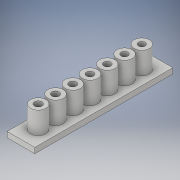
# Autodesk Inventor part: test_gwintow
Saved by Autodesk Inventor 2019 (Build 230136000, 136)
## iProperties
Created: 2019-09-16
Part Number: test_gwintow
Material: Ogólny
Document SubType Name: Modeling
Designer: mikol
Density: 1 g/cm^3
Appearance: Domyślna
Author: mikol
Autodesk Inventor part; units mm, degrees
ref_plane "YZ Plane" through (0, 0, 0) normal (1, 0, 0) x (0, 1, 0)
ref_plane "XZ Plane" through (0, 0, 0) normal (0, 1, 0) x (-1, 0, 0)
ref_plane "XY Plane" through (0, 0, 0) normal (0, 0, 1) x (1, 0, 0)
sketch "Sketch1" plane through (0, 0, 0) normal (0, 1, 0) x (-1, 0, 0)
  line L0 (5, 25) -> (-5, 25)
  line L1 (-5, 25) -> (-5, -25)
  line L2 (-5, -25) -> (5, -25)
  line L3 (5, -25) -> (5, 25)
  line L4 (5, 25) -> (-5, -25) construction
  line L5 (-5, 25) -> (5, -25) construction
  point P0 (0, 0)
  dimension "d0" = 10
  dimension "d1" = 50
  constraints: 12 end point, 2 midpoint, 2 parallel, 1 horizontal, 1 perpendicular
  measures "d0" distance of L2.end L1.end
  measures "d1" distance of L1.end L0.end
extrude "Extrusion1" add sketch "Sketch1" along normal blind 2
sketch "Sketch2" plane through (0, 2, 0) normal (0, 1, 0) x (1, 0, 0)
  circle A0 centre (0, 18.75) radius 1.2
  line L0 (5, 25) -> (-5, 25) projected
  circle A1 centre (0, 12.5) radius 1.225
  circle A2 centre (0, 6.25) radius 1.25
  circle A3 centre (0, 0) radius 1.275
  circle A4 centre (0, -6.25) radius 1.3
  circle A5 centre (0, -12.5) radius 1.325
  circle A6 centre (0, -18.75) radius 1.35
  line L1 (0, 35) -> (0, -35) projected
  line L2 (-5, -25) -> (5, -25) projected
  dimension "d4" = 2.4
  dimension "d5" = 6.25
  dimension "d6" = 2.45
  dimension "d7" = 2.5
  dimension "d8" = 2.55
  dimension "d9" = 2.6
  dimension "d10" = 2.65
  dimension "d11" = 2.7
  dimension "d12" = 6.25
  dimension "d13" = 6.25
  dimension "d14" = 6.25
  dimension "d15" = 6.25
  dimension "d17" = 6.25
  dimension "d18" = 6.25
  dimension "d19" = 6.25
  constraints: 7 centre point, 8 other
  measures "d4" diameter of A0
  measures "d5" distance from line of L0 A0.centre
  measures "d6" diameter of A1
  measures "d7" diameter of A2
  measures "d8" diameter of A3
  measures "d9" diameter of A4
  measures "d10" diameter of A5
  measures "d11" diameter of A6
  measures "d12" distance of A1.centre A0.centre
  measures "d13" distance of A2.centre A1.centre
  measures "d14" distance of A2.centre A3.centre
  measures "d15" distance of A4.centre A3.centre
  measures "d17" distance of A6.centre A5.centre
  measures "d18" distance of A4.centre A5.centre
  measures "d19" distance from line of L2 A6.centre
sketch "Sketch3" plane through (0, 2, 0) normal (0, 1, 0) x (1, 0, 0)
  line L0 (-5, -25) -> (5, -25) projected
  line L1 (5, -25) -> (5, 25) projected
  line L2 (5, 25) -> (-5, 25) projected
  line L3 (-5, 25) -> (-5, -25) projected
  circle A0 centre (0, 18.75) radius 1.2 projected
  circle A1 centre (0, 18.75) radius 2.75
  circle A2 centre (0, 12.5) radius 2.75
  circle A3 centre (0, 6.25) radius 2.75
  circle A4 centre (0, 0) radius 2.75
  circle A5 centre (0, -6.25) radius 2.75
  circle A6 centre (0, -12.5) radius 2.75
  circle A7 centre (0, -18.75) radius 2.75
  dimension "d20" = 5.5
  dimension "d23" = 6.25
  constraints: 7 centre point, 1 coincident, 1 vertical, 12 other
  measures "d20" diameter of A1
  measures "d23" distance of A1.centre A2.centre
extrude "Extrusion2" add sketch "Sketch3" along normal blind 8 contours A0 | A1 | A2 | A3 | A4 | A5 | A6 | A7
extrude "Extrusion3" cut sketch "Sketch2" along normal blind 8
equation "\"d5\" = d19"
equation "\"d12\" = d5"
equation "\"d13\" = d5"
equation "\"d14\" = d5"
equation "\"d15\" = d5"
equation "\"d17\" = d5"
equation "\"d18\" = d5"
body "Solid1"
